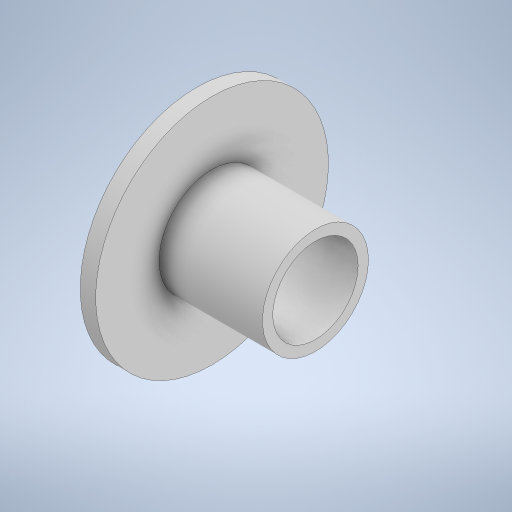
# Autodesk Inventor part: Leg EndCap - ForPoolNoodle
Saved by Autodesk Inventor 2023 (Build 270158000, 158)
## iProperties
Created: 2023-04-05
Part Number: Leg EndCap - ForPoolNoodle
Material: Generic
Document SubType Name: Modeling
Designer: Administrator
Density: 1 g/cm^3
Appearance: Default
Author: Administrator
Autodesk Inventor part; units mm, degrees
ref_plane "YZ Plane" through (0, 0, 0) normal (1, 0, 0) x (0, 1, 0)
ref_plane "XZ Plane" through (0, 0, 0) normal (0, 1, 0) x (-1, 0, 0)
ref_plane "XY Plane" through (0, 0, 0) normal (0, 0, 1) x (1, 0, 0)
sketch "Sketch1" plane through (0, 0, 0) normal (1, 0, 0) x (0, 1, 0)
  circle A0 centre (0, 0) radius 22.5
  dimension "d0" = 45
  constraints: 1 centre point, 1 coincident
  measures "d0" diameter of A0
extrude "Extrusion1" add sketch "Sketch1" along normal blind 3
sketch "Sketch2" plane through (3, 0, 0) normal (1, 0, 0) x (0, 0, -1)
  circle A0 centre (0, 0) radius 10.25
  circle A1 centre (0, 0) radius 8.25
  dimension "d3" = 20.5
  dimension "d4" = 16.5
  constraints: 2 centre point, 2 coincident
  measures "d3" diameter of A0
  measures "d4" diameter of A1
extrude "Extrusion2" add sketch "Sketch2" along normal blind 20
body "Solid1"
